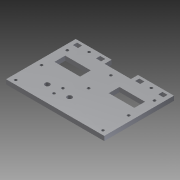
# Autodesk Inventor part: carro x lado polea pieza1
Saved by Autodesk Inventor 2012 (Build 160160000, 160)
## iProperties
Created: 2014-12-16
Part Number: carro x lado polea pieza1
Material: Default
Document SubType Name: Modeling
Designer: PRINCIPAL
Density: 1 g/cm^3
Author: PRINCIPAL
Autodesk Inventor part; units mm, degrees
ref_plane "YZ Plane" through (0, 0, 0) normal (1, 0, 0) x (0, 1, 0)
ref_plane "XZ Plane" through (0, 0, 0) normal (0, 1, 0) x (-1, 0, 0)
ref_plane "XY Plane" through (0, 0, 0) normal (0, 0, 1) x (1, 0, 0)
sketch "Boceto1" plane through (0, 0, 0) normal (0, 0, 1) x (1, 0, 0)
  arc A0 (6, 64.05) -> (4.45, 62.5) centre (6, 62.5) ccw
  arc A1 (4.45, 62.5) -> (6, 60.95) centre (6, 62.5) ccw
  arc A2 (6, 60.95) -> (7.55, 62.5) centre (6, 62.5) ccw
  arc A3 (7.55, 62.5) -> (6, 64.05) centre (6, 62.5) ccw
  arc A4 (55, 64.05) -> (53.45, 62.5) centre (55, 62.5) ccw
  arc A5 (53.45, 62.5) -> (55, 60.95) centre (55, 62.5) ccw
  arc A6 (55, 60.95) -> (56.55, 62.5) centre (55, 62.5) ccw
  arc A7 (56.55, 62.5) -> (55, 64.05) centre (55, 62.5) ccw
  arc A8 (104, 64.05) -> (102.45, 62.5) centre (104, 62.5) ccw
  arc A9 (102.45, 62.5) -> (104, 60.95) centre (104, 62.5) ccw
  arc A10 (104, 60.95) -> (105.55, 62.5) centre (104, 62.5) ccw
  arc A11 (105.55, 62.5) -> (104, 64.05) centre (104, 62.5) ccw
  arc A12 (6, 35.05) -> (4.45, 33.5) centre (6, 33.5) ccw
  arc A13 (4.45, 33.5) -> (6, 31.95) centre (6, 33.5) ccw
  arc A14 (6, 31.95) -> (7.55, 33.5) centre (6, 33.5) ccw
  arc A15 (7.55, 33.5) -> (6, 35.05) centre (6, 33.5) ccw
  arc A16 (55, 39.05) -> (53.45, 37.5) centre (55, 37.5) ccw
  arc A17 (53.45, 37.5) -> (55, 35.95) centre (55, 37.5) ccw
  arc A18 (55, 35.95) -> (56.55, 37.5) centre (55, 37.5) ccw
  arc A19 (56.55, 37.5) -> (55, 39.05) centre (55, 37.5) ccw
  arc A20 (104, 35.05) -> (102.45, 33.5) centre (104, 33.5) ccw
  arc A21 (102.45, 33.5) -> (104, 31.95) centre (104, 33.5) ccw
  arc A22 (104, 31.95) -> (105.55, 33.5) centre (104, 33.5) ccw
  arc A23 (105.55, 33.5) -> (104, 35.05) centre (104, 33.5) ccw
  arc A24 (6, 6.05) -> (4.45, 4.5) centre (6, 4.5) ccw
  arc A25 (4.45, 4.5) -> (6, 2.95) centre (6, 4.5) ccw
  arc A26 (6, 2.95) -> (7.55, 4.5) centre (6, 4.5) ccw
  arc A27 (7.55, 4.5) -> (6, 6.05) centre (6, 4.5) ccw
  arc A28 (104, 6.05) -> (102.45, 4.5) centre (104, 4.5) ccw
  arc A29 (102.45, 4.5) -> (104, 2.95) centre (104, 4.5) ccw
  arc A30 (104, 2.95) -> (105.55, 4.5) centre (104, 4.5) ccw
  arc A31 (105.55, 4.5) -> (104, 6.05) centre (104, 4.5) ccw
  arc A32 (40.5, 24.55) -> (38.95, 23) centre (40.5, 23) ccw
  arc A33 (38.95, 23) -> (40.5, 21.45) centre (40.5, 23) ccw
  arc A34 (40.5, 21.45) -> (42.05, 23) centre (40.5, 23) ccw
  arc A35 (42.05, 23) -> (40.5, 24.55) centre (40.5, 23) ccw
  arc A36 (40.5, 14.55) -> (38.95, 13) centre (40.5, 13) ccw
  arc A37 (38.95, 13) -> (40.5, 11.45) centre (40.5, 13) ccw
  arc A38 (40.5, 11.45) -> (42.05, 13) centre (40.5, 13) ccw
  arc A39 (42.05, 13) -> (40.5, 14.55) centre (40.5, 13) ccw
  arc A40 (20, 74.55) -> (18.45, 73) centre (20, 73) ccw
  arc A41 (18.45, 73) -> (20, 71.45) centre (20, 73) ccw
  arc A42 (20, 71.45) -> (21.55, 73) centre (20, 73) ccw
  arc A43 (21.55, 73) -> (20, 74.55) centre (20, 73) ccw
  arc A44 (90, 74.55) -> (88.45, 73) centre (90, 73) ccw
  arc A45 (88.45, 73) -> (90, 71.45) centre (90, 73) ccw
  arc A46 (90, 71.45) -> (91.55, 73) centre (90, 73) ccw
  arc A47 (91.55, 73) -> (90, 74.55) centre (90, 73) ccw
  line L0 (9.85, 75.35) -> (4.15, 75.35)
  line L1 (4.15, 75.35) -> (4.15, 70.65)
  line L2 (4.15, 70.65) -> (9.85, 70.65)
  line L3 (9.85, 70.65) -> (9.85, 75.35)
  line L4 (35.85, 70.65) -> (35.85, 75.35)
  line L5 (35.85, 75.35) -> (30.15, 75.35)
  line L6 (30.15, 75.35) -> (30.15, 70.65)
  line L7 (30.15, 70.65) -> (35.85, 70.65)
  line L8 (74.15, 70.65) -> (79.85, 70.65)
  line L9 (79.85, 70.65) -> (79.85, 75.35)
  line L10 (79.85, 75.35) -> (74.15, 75.35)
  line L11 (74.15, 75.35) -> (74.15, 70.65)
  line L12 (105.85, 70.65) -> (105.85, 75.35)
  line L13 (105.85, 75.35) -> (100.15, 75.35)
  line L14 (100.15, 75.35) -> (100.15, 70.65)
  line L15 (100.15, 70.65) -> (105.85, 70.65)
  line L16 (38.85, 44) -> (38.85, 56)
  line L17 (38.85, 56) -> (10.15, 56)
  line L18 (10.15, 56) -> (10.15, 44)
  line L19 (10.15, 44) -> (38.85, 44)
  line L20 (71.15, 44) -> (99.85, 44)
  line L21 (99.85, 44) -> (99.85, 56)
  line L22 (99.85, 56) -> (71.15, 56)
  line L23 (71.15, 56) -> (71.15, 44)
  line L24 (-0.2, -0.2) -> (110.2, -0.2)
  line L25 (110.2, -0.2) -> (110.2, 78.2)
  line L26 (110.2, 78.2) -> (69.8, 78.2)
  line L27 (69.8, 78.2) -> (69.8, 70.2)
  line L28 (69.8, 70.2) -> (40.2, 70.2)
  line L29 (40.2, 70.2) -> (40.2, 78.2)
  line L30 (40.2, 78.2) -> (-0.2, 78.2)
  line L31 (-0.2, 78.2) -> (-0.2, -0.2)
  arc A48 (28, 20.75) -> (25.25, 18) centre (28, 18) ccw
  arc A49 (25.25, 18) -> (28, 15.25) centre (28, 18) ccw
  arc A50 (28, 15.25) -> (30.75, 18) centre (28, 18) ccw
  arc A51 (30.75, 18) -> (28, 20.75) centre (28, 18) ccw
  arc A52 (53, 20.75) -> (50.25, 18) centre (53, 18) ccw
  arc A53 (50.25, 18) -> (53, 15.25) centre (53, 18) ccw
  arc A54 (53, 15.25) -> (55.75, 18) centre (53, 18) ccw
  arc A55 (55.75, 18) -> (53, 20.75) centre (53, 18) ccw
  point P0 (0, 0)
  constraints: 112 point on circle, 64 end point, 56 centre point
extrude "Extrusión1" add sketch "Boceto1" along normal blind 5
